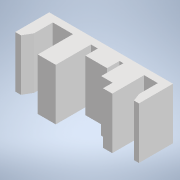
# Autodesk Inventor part: Преобразователь напряжения
Saved by Autodesk Inventor 2021.2 (Build 252289000, 289)
## iProperties
Created: 2021-10-12
Part Number: Преобразователь напряжения
Material: Типовые
Document SubType Name: Modeling
Designer: Surflay
Density: 1 g/cm^3
Appearance: По умолчанию
Author: Surflay
Autodesk Inventor part; units mm, degrees
ref_plane "YZ Plane" through (0, 0, 0) normal (1, 0, 0) x (0, 1, 0)
ref_plane "XZ Plane" through (0, 0, 0) normal (0, 1, 0) x (-1, 0, 0)
ref_plane "XY Plane" through (0, 0, 0) normal (0, 0, 1) x (1, 0, 0)
sketch "Эскиз1" plane through (0, 0, 0) normal (0, 0, 1) x (1, 0, 0)
  line L0 (0, 0) -> (12, 0)
  line L1 (12, 0) -> (12, -5)
  line L2 (12, -5) -> (0, -5)
  line L3 (0, -5) -> (0, 0)
  dimension "d0" = 12
  dimension "d1" = 5
  constraints: 8 end point, 2 parallel, 1 horizontal, 1 perpendicular
  measures "d0" distance of L1.end L2.end
  measures "d1" distance of L0.end L1.end
extrude "Выдавливание1" add sketch "Эскиз1" along normal blind 5
sketch "Эскиз2" plane through (0, -5, 0) normal (0, -1, 0) x (1, 0, 0)
  line L0 (0, 0) -> (0, 5) projected
  line L1 (0, 0.6807) -> (2.9841, 0.6807)
  line L2 (2.9841, 0.6807) -> (2.9841, 4.0939)
  line L3 (2.9841, 4.0939) -> (4.7266, 4.0939)
  line L4 (4.7266, 4.0939) -> (4.7266, 0.6807)
  line L5 (4.7266, 0.6807) -> (5.3913, 0.6807)
  line L6 (5.3913, 0.6807) -> (5.3913, 1.8843)
  line L7 (5.3913, 1.8843) -> (7.493, 1.8843)
  line L8 (7.493, 1.8843) -> (7.493, 0.6807)
  line L9 (7.493, 0.6807) -> (7.8703, 0.6807)
  line L10 (7.8703, 0.6807) -> (7.8703, 2.8364)
  line L11 (7.8703, 2.8364) -> (8.984, 2.8364)
  line L12 (8.984, 2.8364) -> (8.984, 3.7705)
  line L13 (8.984, 3.7705) -> (9.8822, 3.7705)
  line L14 (9.8822, 3.7705) -> (9.8822, 0.6807)
  line L15 (9.8822, 0.6807) -> (11.2116, 0.6807)
  line L16 (11.2116, 0.6807) -> (11.2116, 2.5)
  line L17 (11.2116, 2.5) -> (11.517, 3.3034)
  line L18 (11.517, 3.3034) -> (12, 3.3034)
  line L19 (12, 0) -> (12, 5) projected
  line L20 (0, 0) -> (12, 0) projected
  line L21 (12, 3.3034) -> (12, 0)
  line L22 (12, 0) -> (0, 0)
  line L23 (0, 0.6807) -> (0, 3.3034)
  line L24 (0.559, 3.3034) -> (1.026, 2.5)
  line L25 (1.026, 2.5) -> (1.026, 0.6807)
  line L26 (0.559, 3.3034) -> (0, 3.3034)
  constraints: 48 end point, 15 perpendicular, 10 point on line, 2 vertical, 1 horizontal, 1 parallel
extrude "Выдавливание2" cut sketch "Эскиз2" against normal blind 5 keep common part
